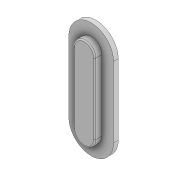
# Autodesk Inventor part: KLEP_KNOPPEN
Saved by Autodesk Inventor 2020.3 (Build 243373000, 373)
## iProperties
Created: 2020-06-10
Part Number: KLEP_KNOPPEN
Material: Generic
Document SubType Name: Modeling
Designer: Gebruiker
Density: 1 g/cm^3
Appearance: Default
Author: Gebruiker
Autodesk Inventor part; units mm, degrees
ref_plane "YZ Plane" through (0, 0, 0) normal (1, 0, 0) x (0, 1, 0)
ref_plane "XZ Plane" through (0, 0, 0) normal (0, 1, 0) x (-1, 0, 0)
ref_plane "XY Plane" through (0, 0, 0) normal (0, 0, 1) x (1, 0, 0)
sketch "Sketch1" plane through (0, 0, 0) normal (0, 0, 1) x (1, 0, 0)
  line L0 (-4.5, 15) -> (4.5, 15)
  line L1 (4.5, 15) -> (4.5, -15)
  line L2 (4.5, -15) -> (-4.5, -15)
  line L3 (-4.5, -15) -> (-4.5, 15)
  line L4 (-4.5, 15) -> (4.5, -15) construction
  line L5 (4.5, 15) -> (-4.5, -15) construction
  circle A0 centre (0, 15) radius 4.5
  circle A1 centre (0, -15) radius 4.5
  point P0 (0, 0)
  point P1 (-4.5, 15)
  point P2 (-4.5, -15)
  dimension "d0" = 9
  dimension "d1" = 30
  constraints: 12 end point, 4 midpoint, 2 parallel, 1 horizontal, 1 perpendicular, 6 other
  measures "d0" distance of L1.end L2.end
  measures "d1" distance of L0.end L1.end
extrude "Extrusion1" add sketch "Sketch1" against normal blind 5
sketch "Sketch3" plane through (0, 0, -5) normal (0, 0, -1) x (-1, 0, 0)
  line L0 (4.5, -15) -> (4.5, 15) projected
  arc A0 (4.5, 15) -> (-4.5, 15) centre (0, 15) ccw projected
  line L1 (-4.5, 15) -> (-4.5, -15) projected
  arc A1 (-4.5, -15) -> (4.5, -15) centre (0, -15) ccw projected
  line L2 (-9.5, -15) -> (-9.5, 15)
  arc A2 (9.5, 15) -> (-9.5, 15) centre (0, 15) ccw
  line L3 (9.5, 15) -> (9.5, -15)
  arc A3 (-9.5, -15) -> (9.5, -15) centre (0, -15) ccw
  point P0 (0, 0)
  dimension "d9" = 5
  constraints: 4 end point, 4 point on circle, 2 centre point, 3 other
  measures "d9" distance between parallel lines of L1 L2
extrude "Extrusion3" add sketch "Sketch3" against normal blind 2
sketch "Sketch5" plane through (0, 0, -5) normal (0, 0, -1) x (-1, 0, 0)
  line L0 (-9.5, 15) -> (-9.5, -15) projected
  arc A0 (-9.5, -15) -> (9.5, -15) centre (0, -15) ccw projected
  line L1 (9.5, -15) -> (9.5, 15) projected
  arc A1 (9.5, 15) -> (-9.5, 15) centre (0, 15) ccw projected
  circle A2 centre (0, 12.9469) radius 1.875
  circle A3 centre (0, -13.0531) radius 1.875
  point P0 (0, 0)
  dimension "d12" = 26
  dimension "d13" = 3.75
  constraints: 2 centre point, 2 vertical alignment, 1 equal radius
  measures "d12" distance of A3.centre A2.centre
  measures "d13" diameter of A2
extrude "Extrusion4" cut sketch "Sketch5" against normal blind 1.8 contours A2 | A3
chamfer "Chamfer1" distance 0.5 angle 45 2 edges at (1.875, 12.9469, -5) (1.875, -13.0531, -5)
fillet "Fillet2" radius 0.5 4 edges at (0, 19.5, 0) (-4.5, 0, 0) (0, -19.5, 0) (4.5, 0, 0)
body "Solid1"
